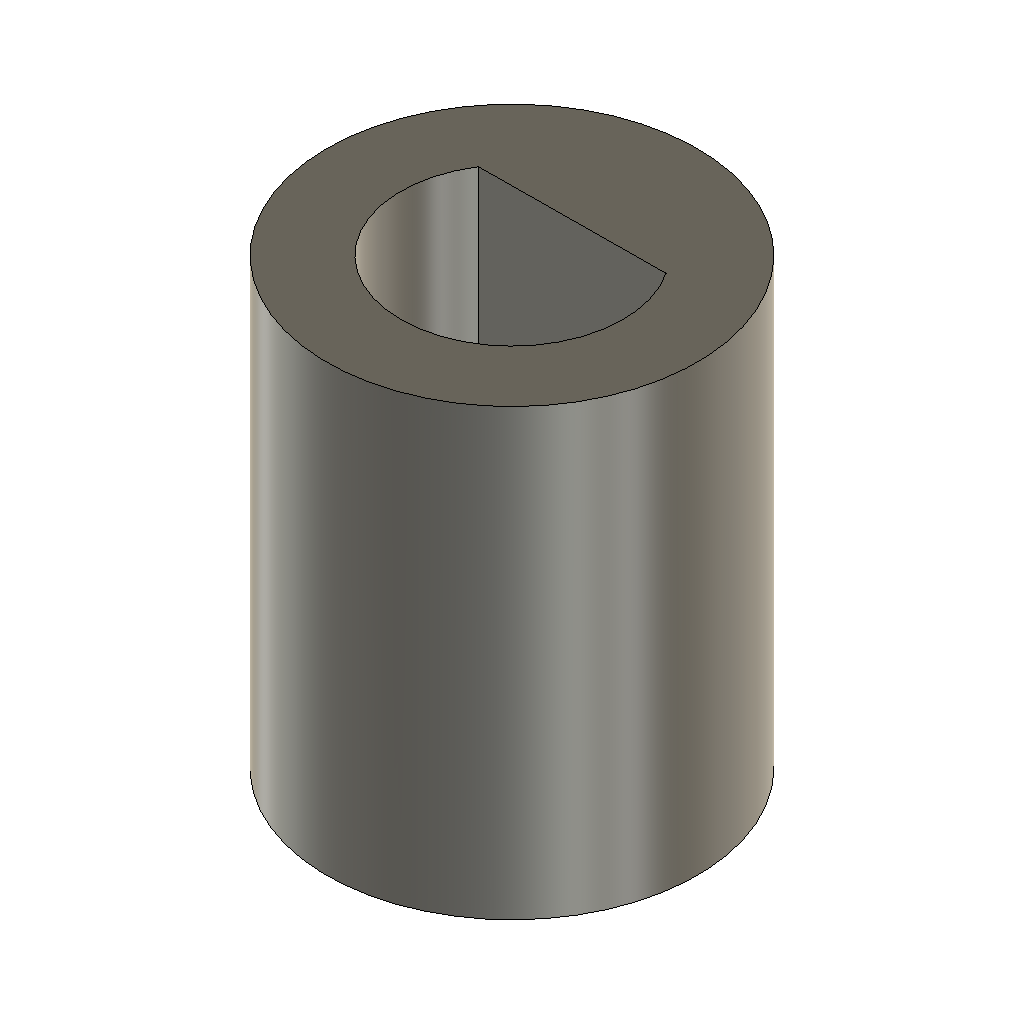
complted (Autodesk Fusion 360 archive; units mm, degrees)
design "3mm too 5mm shaft"
part number: 2026-09-19-16-53-31-621
Autodesk Fusion 360 part; units mm, degrees
note: some values were not read from the file. Set by a fixed rule: which face or edge a step refers to.
sketch "Sketch1" plane through (0, 0, 0) normal (0, 0, 1) x (1, 0, 0)
  circle A0 centre (0, 0) radius 2.5
  dimension "d1" = 5
  constraint coincident A0.centre origin
  measures "d1" diameter of A0
extrude "Extrude1" add sketch "Sketch1" along normal blind 6
sketch "Sketch2" plane through (0, 0, 6) normal (0, 0, 1) x (-1, 0, 0)
  circle A0 centre (0, 0) radius 2.5
  circle A1 centre (0, 0) radius 1.5
  dimension "d4" = 3
  constraint concentric A0 A1
  measures "d4" diameter of A1
extrude "Extrude2" cut sketch "Sketch2" against normal blind 5 contours A1
sketch "Sketch3" plane through (0, 0, 1) normal (0, 0, 1) x (-1, 0, 0)
  circle A0 centre (0, 0) radius 1.5
  line L0 (1.2625, -0.8099) -> (-1.2492, -0.8303)
  arc A1 (0.0066, -1.5) -> (-1.2492, -0.8303) centre (0, 0) ccw
  constraint coincident A0 L0.start
  constraint coincident A0 L0.end
  constraint coincident L0.start A1
  constraint coincident A0 A1.start
extrude "Extrude3" add sketch "Sketch3" along normal blind 5 contours A0 L0 A1 picked at (0.6944, -1.19)

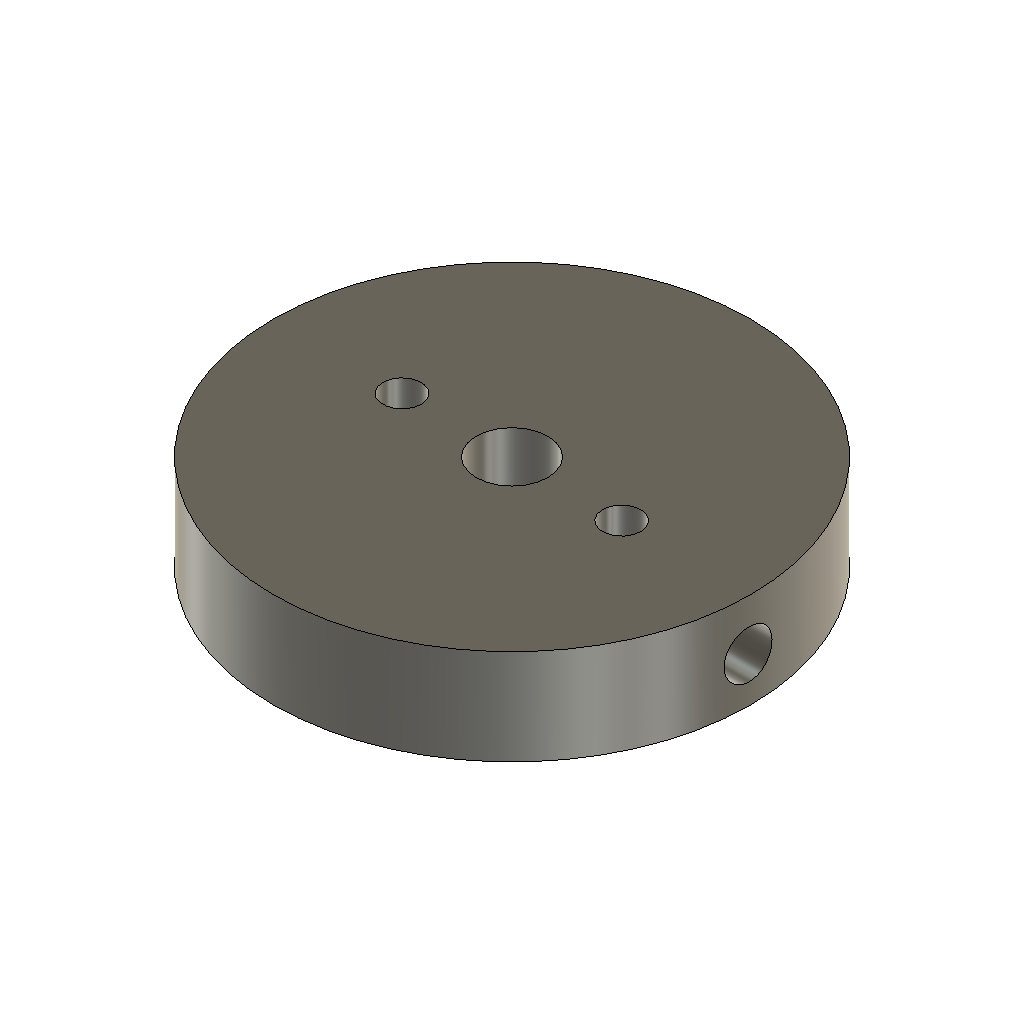
design "frontplate"
part number: 2026-09-10-22-39-12-020
Autodesk Fusion 360 part; units mm, degrees
sketch "Sketch1" plane through (0, 0, 0) normal (0, 0, 1) x (1, 0, 0)
  circle A0 centre (0, 0) radius 10
  dimension "d1" = 20
  constraint coincident A0.centre origin
  measures "d1" diameter of A0
extrude "Extrude1" add sketch "Sketch1" along normal blind 3
sketch "Sketch2" plane through (0, 0, 3) normal (0, 0, 1) x (-1, 0, 0)
  circle A0 centre (0, 0) radius 10
  circle A1 centre (0, 0) radius 1.5
  dimension "d4" = 3
  constraint coincident A0.centre A1.centre
  measures "d4" diameter of A1
extrude "Extrude2" cut sketch "Sketch2" against normal blind 12 contours A1
sketch "Sketch3" plane through (0, 0, 3) normal (0, 0, 1) x (-1, 0, 0)
  circle A0 centre (0, 0) radius 1.5
  circle A1 centre (0, 0) radius 10
  circle A2 centre (-4.6093, 0.0139) radius 0.8
  dimension "d7" = 1.6
  measures "d7" diameter of A2
sketch "Sketch4" plane through (0, 0, 3) normal (0, 0, 1) x (-1, 0, 0)
  circle A0 centre (4.6091, 0) radius 0.8
  dimension "d8" = 1.6
  measures "d8" diameter of A0
extrude "Extrude3" cut sketch "Sketch3" sketch "Sketch4" against normal blind 3 contours A2 of sketch 2
extrude "Extrude4" add 1 faces at (3.3938, 3.5751, 3) along direction (0, 0, 1) blind 17
sketch "Sketch5" plane through (0, 0, 0) normal (1, 0, 0) x (0, 1, 0)
  circle A0 through (0.9391, 6.3685, 6) (-0.5609, 7.2345, 6) (-0.5609, 5.5025, 6)
  dimension "d13" = 2
extrude "Extrude5" cut sketch "Sketch5" along normal blind 5 contours A0 in plane through (6, 0, 0) normal (1, 0, 0)
mirror "Mirror1" about plane through (0, 0, 0) normal (1, 0, 0) of "Extrude5"
extrude "Extrude6" cut 1 faces at (3.3938, 3.5751, 20) along direction (0, 0, -1) blind 9
extrude "Extrude7" cut 1 faces at (3.3938, 3.5751, 11) along direction (0, 0, -1) blind 1.5
extrude "Extrude8" cut 1 faces at (3.3938, 3.5751, 0) along direction (0, 0, 1) blind 1.5
extrude "Extrude9" cut 1 faces at (3.3938, 3.5751, 1.5) along direction (0, 0, 1) blind 3
extrude "Extrude10" cut 1 faces at (3.3938, 3.5751, 9.5) along direction (0, 0, -1) blind 1

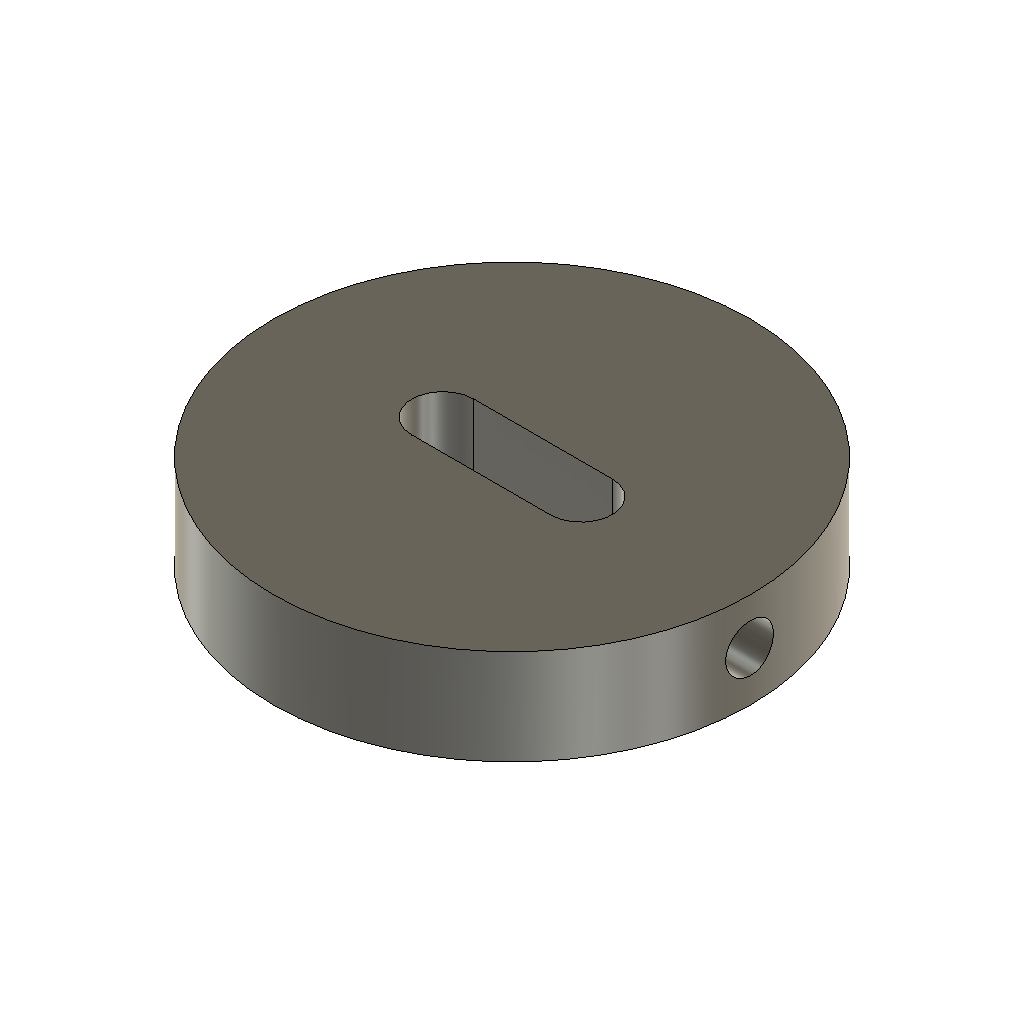
design "backplate"
part number: 2026-09-10-22-58-11-681
Autodesk Fusion 360 part; units mm, degrees
sketch "Sketch1" plane through (0, 0, 0) normal (0, 0, 1) x (1, 0, 0)
  circle A0 centre (0, 0) radius 10
  dimension "d1" = 20
  constraint coincident A0.centre origin
  measures "d1" diameter of A0
extrude "Extrude1" add sketch "Sketch1" along normal blind 3
sketch "Sketch2" plane through (0, 0, 3) normal (0, 0, 1) x (-1, 0, 0)
  circle A0 centre (0, 0) radius 10
  line L0 (-4.2, 1.3) -> (4.2, 1.3)
  line L1 (4.2, 1.3) -> (4.2, -1.3)
  line L2 (4.2, -1.3) -> (-4.2, -1.3)
  line L3 (-4.2, -1.3) -> (-4.2, 1.3)
  line L4 (-4.2, 1.3) -> (4.2, -1.3) construction
  line L5 (4.2, 1.3) -> (-4.2, -1.3) construction
  dimension "d4" = 8.4
  dimension "d5" = 2.6
  constraint horizontal L0
  constraint perpendicular L0 L1
  constraint parallel L0 L2
  constraint parallel L1 L3
  constraint coincident L4 A0.centre
  constraint coincident L5 A0.centre
  constraint coincident A0.centre origin
  measures "d4" distance of L1.end L2.end
  measures "d5" distance of L0.end L1.end
extrude "Extrude2" cut sketch "Sketch2" against normal blind 6 contours L0 L1 L2 L3
fillet "Fillet1" radius 1.3 4 edges at (4.2, 1.3, 1.5) (4.2, -1.3, 1.5) (-4.2, 1.3, 1.5) (-4.2, -1.3, 1.5)
extrude "Extrude3" add 1 faces at (-0.2491, -4.1907, 3) along direction (0, 0, 1) blind 1
hole "Hole1" at (10, 0, 2.0667) direction (-1, 0, 0) diameter 2 depth 4 tip angle 180
mirror "Mirror1" about plane through (0, 0, 0) normal (1, 0, 0) of "Hole1"

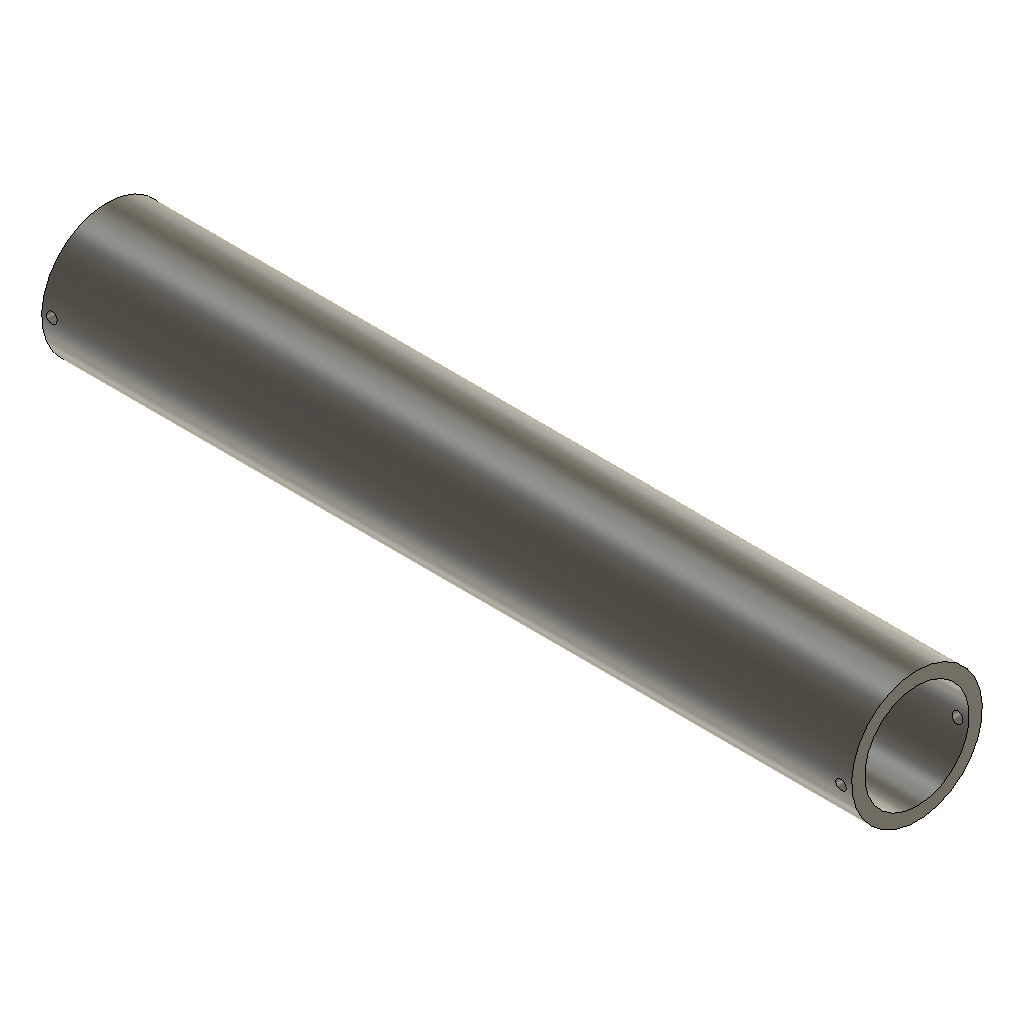
design "handle"
part number: 2026-09-04-00-00-18-277
Autodesk Fusion 360 part; units mm, degrees
sketch "Sketch2" plane through (0, 0, 0) normal (0, 0, 1) x (1, 0, 0)
  circle A0 centre (0, 0) radius 10.5
  dimension "d15" = 21
  constraint coincident A0.centre origin
  measures "d15" diameter of A0
extrude "Extrude3" add sketch "Sketch2" along normal blind 100
extrude "Extrude4" add 1 faces at (-2.9623, 1.0316, 100) along direction (0, 0, 1) blind 55
shell "Shell4" thickness 0.5 removed faces 1 at (-2.9623, 1.0316, 155)
sketch "Sketch3" plane through (0, 0, 0) normal (0, 1, 0) x (1, 0, 0)
  line L0 (1.8551, -103.1591) -> (-4.1449, -103.1591)
  line L1 (-4.1449, -103.1591) -> (-4.1449, -77.5591)
  line L2 (-4.1449, -77.5591) -> (1.8551, -77.5591)
  line L3 (1.8551, -77.5591) -> (1.8551, -103.1591)
  dimension "d21" = 6
  dimension "d22" = 25.6
  constraint horizontal L0
  constraint vertical L1
  constraint horizontal L2
  constraint vertical L3
  measures "d21" distance of L0.start L0.end
  measures "d22" distance of L0.start L2.end
extrude "Extrude5" cut sketch "Sketch3" along normal blind 19
move_body "Move1" bodies 1 to x (0, 0, -1) y (0, 1, 0) z (1, 0, 0) at (-77.5, 0, 77.5)
extrude "Extrude6" cut 1 faces at (-77, 3.5886, 75.2736) along direction (-1, 0, 0) blind 1
sketch "Sketch4" plane through (0, 0, 0) normal (0, 1, 0) x (1, 0, 0)
  circle A0 centre (75.3676, -76.1708) radius 1
  dimension "d27" = 2
  measures "d27" diameter of A0
extrude "Extrude7" cut sketch "Sketch4" along normal blind 21
mirror "Mirror1" about plane through (0, 0, 0) normal (0, 1, 0) of "Extrude7"
sketch "Sketch5" plane through (0, 0, 0) normal (0, 1, 0) x (1, 0, 0)
  circle A0 centre (-75.5671, -78.134) radius 1
  dimension "d32" = 2
  measures "d32" diameter of A0
extrude "Extrude8" cut sketch "Sketch5" along normal blind 19
mirror "Mirror2" about plane through (0, 0, 0) normal (0, 1, 0) of "Extrude8"
move_face "OffsetFaces1" offset 2 1 faces at (0.0197, 10.0042, 74.3115)
